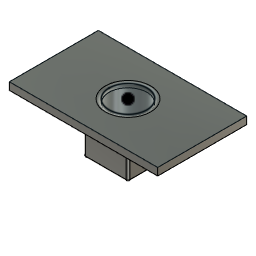
Power LED Holder v8 (Autodesk Fusion 360 design; units mm, degrees)
Autodesk Fusion 360 part; units mm, degrees
sketch "Sketch2" plane through (0, 0, 0) normal (0, 0, 1) x (1, 0, 0)
  line L0 (3, -3) -> (-3, -3)
  line L1 (-3, -3) -> (-3, 3)
  line L2 (-3, 3) -> (3, 3)
  line L3 (3, 3) -> (3, -3)
  line L4 (3, -3) -> (-3, 3) construction
  line L5 (-3, -3) -> (3, 3) construction
  dimension "d1" = 6
  dimension "d2" = 6
  constraint horizontal L0
  constraint perpendicular L0 L1
  constraint parallel L0 L2
  constraint parallel L1 L3
  constraint coincident L4 origin
  constraint coincident L5 origin
  measures "d1" distance of L1.end L2.end
  measures "d2" distance of L0.end L1.end
extrude "Extrude1" add sketch "Sketch2" along normal blind 5.8
sketch "Sketch3" plane through (0, 0, 5.8) normal (0, 0, 1) x (-1, 0, 0)
  line L0 (-3, -3) -> (3, -3)
  line L1 (3, -3) -> (3, 3)
  line L2 (3, 3) -> (-3, 3)
  line L3 (-3, 3) -> (-3, -3)
  line L4 (10, 6) -> (-10, 6)
  line L5 (-10, 6) -> (-10, -6)
  line L6 (-10, -6) -> (10, -6)
  line L7 (10, -6) -> (10, 6)
  dimension "d17" = 20
  dimension "d18" = 10
  dimension "d19" = 12
  dimension "d20" = 6
  constraint horizontal L4
  constraint perpendicular L4 L5
  constraint perpendicular L6 L7
  constraint perpendicular L5 L6
  measures "d17" distance of L5.end L6.end
  measures "d18" distance of origin L7
  measures "d19" distance of L4.start L6.end
  measures "d20" distance of origin L4
extrude "Extrude2" add sketch "Sketch3" along normal blind 1 contours L0 L1 L2 L3 | L4 L5 L6 L7
fillet "Fillet1" radius 0.25 8 edges at (0, -3, 0) (3, -3, 2.9) (3, 0, 0) (3, 3, 2.9) (0, 3, 0) (-3, 0, 0) (-3, -3, 2.9) (-3, 3, 2.9)
sketch "Sketch4" plane through (0, 0, 6.8) normal (0, 0, 1) x (-1, 0, 0)
  line L0 (10, -6) -> (10, 6)
  line L1 (10, 6) -> (-10, 6)
  line L2 (-10, 6) -> (-10, -6)
  line L3 (-10, -6) -> (10, -6)
  circle A0 centre (0, 0) radius 2.55
  dimension "d10" = 5.1
  constraint coincident A0.centre origin
  measures "d10" diameter of A0
extrude "Extrude3" cut sketch "Sketch4" against normal blind 6 contours A0
fillet "Fillet2" radius 1 1 edges at (2.3774, -0.9221, 0.8)
fillet "Fillet3" radius 0.5 1 edges at (2.3774, -0.9221, 6.8)
equation "d2 = d1"
equation "d18 = d17 / 2"
equation "d20 = d19 / 2"
